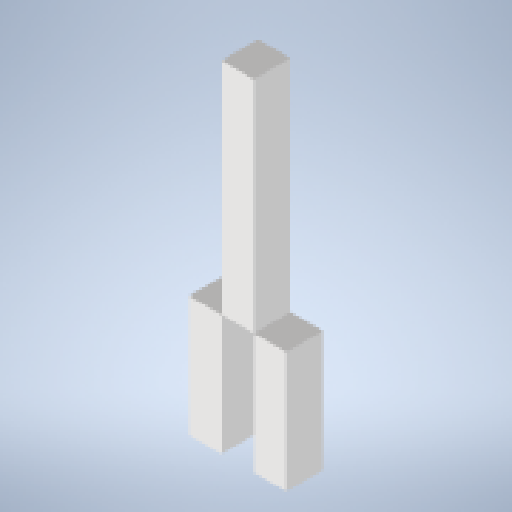
# Autodesk Inventor part: ForearmActuatorConnectorBoundingBox
Saved by Autodesk Inventor 2023 (Build 270158000, 158)
## iProperties
Created: 2023-03-28
Part Number: ForearmActuatorConnectorBoundingBox
Material: Generic
Document SubType Name: Modeling
Designer: LattePanda
Density: 1 g/cm^3
Appearance: Default
Author: LattePanda
Autodesk Inventor part; units mm, degrees
ref_plane "YZ Plane" through (0, 0, 0) normal (1, 0, 0) x (0, 1, 0)
ref_plane "XZ Plane" through (0, 0, 0) normal (0, 1, 0) x (-1, 0, 0)
sketch "Sketch1" plane through (0, 0, 0) normal (0, 0, 1) x (1, 0, 0)
  line L0 (-2.81, 5) -> (2.81, 5)
  line L1 (2.81, 5) -> (2.81, -33.1)
  line L2 (2.81, -33.1) -> (-2.81, -33.1)
  line L3 (-2.81, -33.1) -> (-2.81, 5)
  line L4 (-2.81, -33.1) -> (-8.43, -33.1)
  line L5 (-8.43, -33.1) -> (-8.43, -54)
  line L6 (-8.43, -54) -> (-2.81, -54)
  line L7 (-2.81, -54) -> (-2.81, -33.1)
  line L8 (-3.81, 1) -> (-3.81, -16.3736) construction
  line L9 (3.81, -16.3736) -> (3.81, 1) construction
  line L10 (-0.64, 6) -> (-3.81, 6) construction
  line L11 (-9.398, -55) -> (-6.228, -55) projected
  line L12 (0, -67.2) -> (0, 18.2) construction
  line L13 (2.81, -33.1) -> (8.43, -33.1)
  line L14 (8.43, -33.1) -> (8.43, -54)
  line L15 (8.43, -54) -> (2.81, -54)
  line L16 (2.81, -54) -> (2.81, -33.1)
  point P0 (0, 0)
  point P1 (-7.813, -55)
  dimension "d0" = 1
  dimension "d1" = 1
  dimension "d2" = 1
  dimension "d3" = 38.1
  dimension "d4" = 1
  constraints: 24 end point, 4 parallel, 3 symmetric about line, 2 horizontal, 2 perpendicular, 1 collinear, 1 midpoint
  measures "d0" distance between parallel lines of L8 L3
  measures "d1" distance between parallel lines of L9 L1
  measures "d2" distance between parallel lines of L10 L0
  measures "d3" distance of L2.end L0.start
  measures "d4" distance from line of point (-7.813, -55) L6
ref_plane "Work Plane1" through (6.228, -54, -6.35) normal (0, 0, -1) x (0, 1, 0)
extrude "Extrusion1" add sketch "Sketch1" against normal up to surface (6.35 mm away)
body "Solid1"
